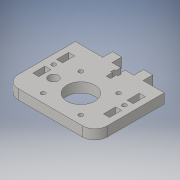
# Autodesk Inventor part: A8-0002
Saved by Autodesk Inventor 2016 SP2 (Build 200236200, 236)
## iProperties
Created: 2017-04-22
Part Number: A8-0002
Material: Generic
Document SubType Name: Modeling
Designer: EV
Density: 1 g/cm^3
Appearance: Default
Author: EV
Autodesk Inventor part; units mm, degrees
ref_plane "YZ Plane" through (0, 0, 0) normal (1, 0, 0) x (0, 1, 0)
sketch "Sketch1" plane through (0, 0, 0) normal (0, 1, 0) x (-1, 0, 0)
  line L0 (-10, 0) -> (-63, 0)
  line L1 (-73, -10) -> (-73, -57)
  line L2 (0, -57) -> (0, -10)
  line L3 (-22.5, -57) -> (-22.5, -65)
  line L4 (-22.5, -65) -> (-30, -65)
  line L5 (-30, -65) -> (-30, -57)
  line L6 (-48, -57) -> (-48, -65)
  line L7 (-48, -65) -> (-55.5, -65)
  line L8 (-55.5, -65) -> (-55.5, -57)
  line L9 (-73, -57) -> (-55.5, -57)
  line L10 (-22.5, -57) -> (0, -57)
  line L11 (-37.25, -57) -> (-37.25, -53)
  line L12 (-37.25, -53) -> (-36, -53)
  line L13 (-36, -53) -> (-36, -50)
  line L14 (-36, -50) -> (-37.25, -50)
  line L15 (-37.25, -50) -> (-37.25, -45)
  line L16 (-37.25, -45) -> (-40.75, -45)
  line L17 (-40.75, -45) -> (-40.75, -50)
  line L18 (-40.75, -50) -> (-42, -50)
  line L19 (-42, -50) -> (-42, -53)
  line L20 (-42, -53) -> (-40.75, -53)
  line L21 (-40.75, -53) -> (-40.75, -57)
  line L22 (-48, -57) -> (-40.75, -57)
  line L23 (-37.25, -57) -> (-30, -57)
  arc A0 (0, -10) -> (-10, 0) centre (-10, -10) ccw
  arc A1 (-63, 0) -> (-73, -10) centre (-63, -10) ccw
  line L24 (-5, -17) -> (-10, -17)
  line L25 (-10, -17) -> (-10, -27)
  line L26 (-10, -27) -> (-5, -27)
  line L27 (-5, -27) -> (-5, -17)
  line L28 (-5, -36.5) -> (-10, -36.5)
  line L29 (-10, -36.5) -> (-10, -46.5)
  line L30 (-10, -46.5) -> (-5, -46.5)
  line L31 (-5, -46.5) -> (-5, -36.5)
  line L32 (-63, -17) -> (-68, -17)
  line L33 (-68, -17) -> (-68, -27)
  line L34 (-68, -27) -> (-63, -27)
  line L35 (-63, -27) -> (-63, -17)
  line L36 (-63, -36.5) -> (-68, -36.5)
  line L37 (-68, -36.5) -> (-68, -46.5)
  line L38 (-68, -46.5) -> (-63, -46.5)
  line L39 (-63, -46.5) -> (-63, -36.5)
  line L40 (-39, -45) -> (-39, -65) construction
  point P0 (0, 0)
  point P1 (-73, 0)
  dimension "d0" = 73
  dimension "d1" = 57
  dimension "d2" = 22.5
  dimension "d3" = 7.5
  dimension "d4" = 8
  dimension "d5" = 17.5
  dimension "d6" = 18
  dimension "d7" = 3.5
  dimension "d8" = 6
  dimension "d9" = 4
  dimension "d10" = 3
  dimension "d11" = 5
  dimension "d12" = 10
  dimension "d13" = 5
  dimension "d14" = 10
  dimension "d15" = 5
  dimension "d17" = 9.5
  dimension "d18" = 5
  dimension "d19" = 10.5
  constraints: 82 end point, 26 perpendicular, 14 point on line, 13 parallel, 9 equal length, 8 collinear, 5 horizontal, 4 point on circle, 4 tangent, 2 centre point, 1 equal radius, 1 midpoint, 1 vertical
  measures "d0" distance of point (0, 0) point (-73, 0)
  measures "d1" distance of L2.start point (0, 0)
  measures "d2" distance between parallel lines of L2 L3
  measures "d3" distance of L3.end L4.end
  measures "d4" distance of L3.start L3.end
  measures "d5" distance between parallel lines of L1 L8
  measures "d6" distance between parallel lines of L5 L6
  measures "d7" distance between parallel lines of L21 L11
  measures "d8" distance between parallel lines of L13 L19
  measures "d9" distance of L20.end L21.end
  measures "d10" distance of L18.end L19.end
  measures "d11" distance of L16.end L17.end
  measures "d12" radius of A0
  measures "d13" distance of L24.start L24.end
  measures "d14" distance of L26.end L24.start
  measures "d15" distance between parallel lines of L2 L27
  measures "d17" distance between parallel lines of L26 L28
  measures "d18" distance between parallel lines of L1 L33
  measures "d19" distance between parallel lines of L10 L30
extrude "Extrusion1" add sketch "Sketch1" along normal blind 8
sketch "Sketch2" plane through (0, 8, 0) normal (0, 1, 0) x (1, 0, 0)
  line L0 (63, 36.5) -> (63, 46.5) construction
  line L1 (63, 46.5) -> (68, 46.5) construction
  line L2 (68, 46.5) -> (68, 36.5) construction
  line L3 (68, 36.5) -> (63, 36.5) construction
  line L4 (63, 17) -> (63, 27) construction
  line L5 (63, 27) -> (68, 27) construction
  line L6 (68, 27) -> (68, 17) construction
  line L7 (68, 17) -> (63, 17) construction
  line L8 (5, 36.5) -> (5, 46.5) construction
  line L9 (5, 46.5) -> (10, 46.5) construction
  line L10 (10, 46.5) -> (10, 36.5) construction
  line L11 (10, 36.5) -> (5, 36.5) construction
  line L12 (5, 17) -> (5, 27) construction
  line L13 (5, 27) -> (10, 27) construction
  line L14 (10, 27) -> (10, 17) construction
  line L15 (10, 17) -> (5, 17) construction
  line L16 (73, 10) -> (73, 57) construction
  line L17 (73, 57) -> (55.5, 57) construction
  line L18 (55.5, 57) -> (55.5, 65) construction
  line L19 (55.5, 65) -> (48, 65) construction
  line L20 (48, 65) -> (48, 57) construction
  line L21 (48, 57) -> (40.75, 57) construction
  line L22 (40.75, 57) -> (40.75, 53) construction
  line L23 (40.75, 53) -> (42, 53) construction
  line L24 (42, 53) -> (42, 50) construction
  line L25 (42, 50) -> (40.75, 50) construction
  line L26 (40.75, 50) -> (40.75, 45) construction
  line L27 (40.75, 45) -> (37.25, 45) construction
  line L28 (37.25, 45) -> (37.25, 50) construction
  line L29 (37.25, 50) -> (36, 50) construction
  line L30 (36, 50) -> (36, 53) construction
  line L31 (36, 53) -> (37.25, 53) construction
  line L32 (37.25, 53) -> (37.25, 57) construction
  line L33 (37.25, 57) -> (30, 57) construction
  line L34 (30, 57) -> (30, 65) construction
  line L35 (30, 65) -> (22.5, 65) construction
  line L36 (22.5, 65) -> (22.5, 57) construction
  line L37 (22.5, 57) -> (0, 57) construction
  line L38 (0, 57) -> (0, 10) construction
  arc A0 (0, 10) -> (10, 0) centre (10, 10) ccw construction
  line L39 (10, 0) -> (63, 0) construction
  arc A1 (63, 0) -> (73, 10) centre (63, 10) ccw construction
  line L40 (10, 27) -> (5, 27) construction
  line L41 (7.5, 27) -> (7.5, 36.5) construction
  line L42 (5, 36.5) -> (10, 36.5) construction
  line L43 (65.5, 27) -> (65.5, 36.5) construction
  line L44 (68, 36.5) -> (63, 36.5) construction
  line L45 (23.5, 38) -> (54.5, 38) construction
  line L46 (54.5, 38) -> (54.5, 7) construction
  line L47 (54.5, 7) -> (23.5, 7) construction
  line L48 (23.5, 7) -> (23.5, 38) construction
  line L49 (23.5, 22.5) -> (54.5, 22.5) construction
  point P0 (0, 0)
  point P1 (7.5, 31.75)
  point P2 (65.5, 31.75)
  point P3 (17, 22)
  point P4 (39, 22.5)
  dimension "d22" = 31
  dimension "d23" = 31
  dimension "d24" = 7
  dimension "d25" = 23.5
  dimension "d26" = 17
  dimension "d27" = 22
  constraints: 14 end point, 9 midpoint, 4 coincident, 2 parallel, 1 horizontal, 1 perpendicular
  measures "d22" distance between parallel lines of L46 L48
  measures "d23" distance of L47.end L45.start
  measures "d24" distance between parallel lines of L39 L47
  measures "d25" distance between parallel lines of L38 L48
  measures "d26" distance from line of L38 point (17, 22)
  measures "d27" distance from line of point (17, 22) L39
hole "Hole1" at (7.5, 8, -31.75) at (65.5, 8, -31.75) at (23.5, 8, -38) at (54.5, 8, -38) at (54.5, 8, -7) at (23.5, 8, -7) direction (0, -1, 0) diameter 3.5 end through all
hole "Hole2" at (17, 8, -22) direction (0, -1, 0) diameter 8 end through all
hole "Hole3" at (39, 8, -22.5) direction (0, -1, 0) diameter 23 end through all
ref_plane "Work Plane1" through (0, 4, 0) normal (0, 1, 0) x (-1, 0, 0)
ref_plane "Work Plane2" through (39, 0, -45) normal (1, 0, 0) x (0, 0, -1)
equation "\"d49\" = 0.5 * THICKNESS"
equation "\"THICKNESS\" = 8"
body "Solid1"
